Directional Motor Fixation (Autodesk Fusion 360 design; units mm, degrees)
Autodesk Fusion 360 part; units mm, degrees
sketch "Sketch1" plane through (0, 0, 0) normal (0, 0, 1) x (1, 0, 0)
  line L0 (20.5, -4) -> (-20.5, -4)
  line L1 (-20.5, -4) -> (-20.5, 4)
  line L2 (-20.5, 4) -> (20.5, 4)
  line L3 (20.5, 4) -> (20.5, -4)
  line L4 (20.5, -4) -> (-20.5, 4) construction
  line L5 (-20.5, -4) -> (20.5, 4) construction
  line L6 (-16, 0) -> (16, 0) construction
  circle A0 centre (-16, 0) radius 2.15
  circle A1 centre (16, 0) radius 2.15
  dimension "d1" = 8
  dimension "d2" = 41
  dimension "d3" = 32
  dimension "d4" = 4.3
  dimension "d5" = 4.3
  constraint perpendicular L0 L1
  constraint parallel L0 L2
  constraint parallel L1 L3
  constraint horizontal L0
  constraint coincident L4 origin
  constraint coincident L5 origin
  constraint parallel L2 L6
  constraint midpoint origin L6
  constraint coincident L6.start A0.centre
  constraint coincident L6.end A1.centre
  measures "d1" distance of L0.end L1.end
  measures "d2" distance of L1.end L2.end
  measures "d3" distance of L6.start L6.end
  measures "d4" diameter of A0
  measures "d5" diameter of A1
extrude "Extrude1" add sketch "Sketch1" along normal blind 13
sketch "Sketch3" plane through (0, 0, 0) normal (0, 0, -1) x (1, 0, 0)
  circle A0 centre (16, 0) radius 2.15
  circle A1 centre (-16, 0) radius 2.15
  line L0 (-20.5, -4) -> (20.5, -4)
  line L1 (20.5, -4) -> (20.5, 4)
  line L2 (20.5, 4) -> (-20.5, 4)
  line L3 (-20.5, 4) -> (-20.5, -4)
  line L4 (12, -4) -> (-12, -4)
  line L5 (-12, -4) -> (-12, 4)
  line L6 (-12, 4) -> (12, 4)
  line L7 (12, 4) -> (12, -4)
  line L8 (12, -4) -> (-12, 4) construction
  line L9 (-12, -4) -> (12, 4) construction
  dimension "d9" = 24
  constraint perpendicular L4 L5
  constraint parallel L4 L6
  constraint parallel L5 L7
  constraint horizontal L4
  constraint coincident L8 origin
  constraint coincident L9 origin
  constraint coincident L0 L4.start
  measures "d9" distance of L5.end L6.end
extrude "Extrude2" cut sketch "Sketch3" against normal blind 9.5 contours L0 L2 L4 L5 L6 L7
